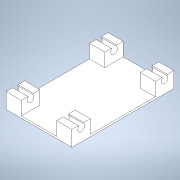
# Autodesk Inventor part: Kuka_base
Saved by Autodesk Inventor 2022 (Build 260153000, 153)
## iProperties
Created: 2022-08-12
Part Number: Kuka_base
Material: Generic
Document SubType Name: Modeling
Designer: Alok
Density: 1 g/cm^3
Appearance: Default
Author: Alok
Autodesk Inventor part; units mm, degrees
ref_plane "YZ Plane" through (0, 0, 0) normal (1, 0, 0) x (0, 1, 0)
ref_plane "XZ Plane" through (0, 0, 0) normal (0, 1, 0) x (-1, 0, 0)
ref_plane "XY Plane" through (0, 0, 0) normal (0, 0, 1) x (1, 0, 0)
sketch "Sketch1" plane through (0, 0, 0) normal (0, 1, 0) x (-1, 0, 0)
  line L0 (195, 302.5) -> (-195, 302.5)
  line L1 (-195, 302.5) -> (-195, -302.5)
  line L2 (-195, -302.5) -> (195, -302.5)
  line L3 (195, -302.5) -> (195, 302.5)
  line L4 (195, 302.5) -> (-195, -302.5) construction
  line L5 (-195, 302.5) -> (195, -302.5) construction
  point P0 (0, 0)
  dimension "d0" = 390
  dimension "d1" = 605
  constraints: 12 end point, 2 midpoint, 2 parallel, 1 horizontal, 1 perpendicular
  measures "d0" distance of L2.end L1.end
  measures "d1" distance of L1.end L0.end
extrude "Extrusion1" add sketch "Sketch1" along normal blind 12
sketch "Sketch2" plane through (0, 12, 0) normal (0, 1, 0) x (1, 0, 0)
  line L0 (-195, 302.5) -> (-195, -302.5) projected
  line L1 (-195, -302.5) -> (-195, -192.5)
  line L2 (-195, -302.5) -> (-85, -302.5) construction
  line L3 (-195, -192.5) -> (-105, -192.5)
  line L4 (-105, -192.5) -> (-105, -302.5)
  line L5 (-105, -302.5) -> (-195, -302.5)
  point P0 (0, 0)
  dimension "d4" = 110
  dimension "d5" = 90
  dimension "d6" = 90
  dimension "d7" = 90
  constraints: 10 end point, 4 perpendicular, 1 collinear, 1 horizontal
  measures "d4" distance of L0.end L1.end
  measures "d5" angle of L2 L1
  measures "d6" distance of L1.end L3.end
  measures "d7" angle of L1 L3
extrude "Extrusion2" add sketch "Sketch2" along normal blind 80
sketch "Sketch3" plane through (-195, 0, -302.5) normal (-1, 0, 0) x (0, 0, 1)
  line L0 (495, 92) -> (605, 92) projected
  line L1 (495, 92) -> (550, 92)
  line L2 (550, 92) -> (550, 73)
  line L3 (550, 92) -> (569, 92) construction
  circle A0 centre (550, 73) radius 20
  point P0 (302.5, 0)
  point P1 (543.755, 92)
  point P2 (556.245, 92)
  dimension "d10" = 55
  dimension "d11" = 19
  dimension "d12" = 90
  dimension "d13" = 40
  constraints: 6 end point, 1 centre point, 1 coincident, 1 horizontal, 1 midpoint, 1 perpendicular, 1 vertical
  measures "d10" distance of L0.start L1.end
  measures "d11" distance of L1.end L2.end
  measures "d12" angle of L2 L3
  measures "d13" diameter of A0
extrude "Extrusion3" cut sketch "Sketch3" against normal blind 110 contours L0 A0 picked at (549.7853, 66.101)
sketch "Sketch4" plane through (-195, 0, -302.5) normal (-1, 0, 0) x (0, 0, 1)
  line L0 (495, 92) -> (543.755, 92) projected
  line L1 (543.755, 92) -> (533.755, 92)
  line L2 (533.755, 92) -> (537.2905, 88.4645)
  arc A0 (543.755, 92) -> (556.245, 92) centre (550, 73) ccw projected
  line L3 (537.2905, 88.4645) -> (543.755, 92)
  point P0 (302.5, 0)
  dimension "d16" = 10
  dimension "d17" = 5
  dimension "d18" = 45
  constraints: 6 end point, 1 point on line
  measures "d16" distance of L0.end L1.end
  measures "d17" distance of L1.end L2.end
  measures "d18" angle of L2 L1
extrude "Extrusion4" cut sketch "Sketch4" against normal blind 110
sketch "Sketch5" plane through (-195, 0, -302.5) normal (-1, 0, 0) x (0, 0, 1)
  arc A0 (537.3715, 88.5088) -> (556.245, 92) centre (550, 73) ccw projected
  line L0 (556.245, 92) -> (566.245, 92)
  line L1 (556.245, 92) -> (605, 92) projected
  line L2 (556.245, 92) -> (566.245, 92) construction
  line L3 (566.245, 92) -> (562.7095, 88.4645)
  line L4 (562.7095, 88.4645) -> (556.245, 92)
  point P0 (302.5, 0)
  dimension "d21" = 10
  dimension "d22" = 0
  dimension "d23" = 5
  dimension "d24" = 45
  constraints: 8 end point, 2 collinear, 1 horizontal
  measures "d21" distance of L0.start L0.end
  measures "d22" distance between parallel lines of L0 L2
  measures "d23" distance of L0.end L3.end
  measures "d24" angle of L0 L3
extrude "Extrusion5" cut sketch "Sketch5" against normal blind 110
mirror "Mirror1" about plane through (0, 0, 0) normal (0, 0, 1) of "Extrusion2"
sketch "Sketch6" plane through (-105, 12, -302.5) normal (1, 0, 0) x (0, 0, -1)
  line L0 (-110, 80) -> (-55, 80)
  line L1 (0, 80) -> (-110, 80) projected
  line L2 (-55, 80) -> (-55, 61)
  circle A0 centre (-55, 61) radius 20
  point P0 (-302.5, -12)
  point P1 (-61.245, 80)
  point P2 (-48.755, 80)
  dimension "d27" = 55
  dimension "d28" = 19
  dimension "d29" = 40
  constraints: 4 end point, 1 centre point, 1 coincident, 1 midpoint, 1 vertical
  measures "d27" distance of L0.start L0.end
  measures "d28" distance of L0.end L2.end
  measures "d29" diameter of A0
extrude "Extrusion6" cut sketch "Sketch6" against normal blind 110 contours L0 L1 A0 picked at (-55.2147, 54.101)
mirror "Mirror2" about plane through (0, 0, 0) normal (1, 0, 0) of "Extrusion2", "Mirror1"
sketch "Sketch7" plane through (195, 0, 302.5) normal (1, 0, 0) x (0, 0, -1)
  arc A0 (543.755, 92) -> (556.245, 92) centre (550, 73) ccw projected
  circle A1 centre (550, 73) radius 20
  point P0 (302.5, 0)
  constraints: 1 centre point, 1 coincident
extrude "Extrusion7" cut sketch "Sketch7" against normal blind 110
sketch "Sketch8" plane through (195, 0, 302.5) normal (1, 0, 0) x (0, 0, -1)
  arc A0 (42.3715, 88.5088) -> (67.6285, 88.5088) centre (55, 73) ccw projected
  circle A1 centre (55, 73) radius 20
  point P0 (302.5, 0)
  point P1 (67.6285, 88.5088)
  constraints: 1 centre point, 1 coincident
extrude "Extrusion8" cut sketch "Sketch8" against normal blind 110
sketch "Sketch9" plane through (195, 0, 302.5) normal (1, 0, 0) x (0, 0, -1)
  line L0 (48.755, 92) -> (38.755, 92)
  line L1 (48.755, 92) -> (0, 92) projected
  line L2 (38.755, 92) -> (42.3026, 88.4524)
  arc A0 (48.755, 92) -> (61.245, 92) centre (55, 73) ccw projected
  line L3 (42.3026, 88.4524) -> (48.755, 92)
  point P0 (302.5, 0)
  dimension "d36" = 10
  dimension "d37" = 45
  constraints: 6 end point, 1 point on circle, 1 point on line
  measures "d36" distance of L0.start L0.end
  measures "d37" angle of L2 L0
extrude "Extrusion9" cut sketch "Sketch9" against normal blind 110
sketch "Sketch10" plane through (195, 0, 302.5) normal (1, 0, 0) x (0, 0, -1)
  arc A0 (42.3026, 88.4524) -> (61.245, 92) centre (55, 73) ccw projected
  line L0 (61.245, 92) -> (71.245, 92)
  line L1 (110, 92) -> (61.245, 92) projected
  line L2 (71.245, 92) -> (67.7095, 88.4645)
  line L3 (67.7095, 88.4645) -> (61.245, 92)
  point P0 (302.5, 0)
  dimension "d40" = 10
  dimension "d41" = 5
  dimension "d42" = 45
  constraints: 6 end point, 1 point on line
  measures "d40" distance of L0.start L0.end
  measures "d41" distance of L0.end L2.end
  measures "d42" angle of L0 L2
extrude "Extrusion10" cut sketch "Sketch10" against normal blind 110
sketch "Sketch11" plane through (195, 0, 302.5) normal (1, 0, 0) x (0, 0, -1)
  line L0 (543.755, 92) -> (495, 92) projected
  line L1 (543.755, 92) -> (533.755, 92)
  line L2 (533.755, 92) -> (537.2905, 88.4645)
  arc A0 (543.755, 92) -> (556.245, 92) centre (550, 73) ccw projected
  line L3 (537.2905, 88.4645) -> (543.755, 92)
  point P0 (302.5, 0)
  dimension "d45" = 10
  dimension "d46" = 5
  dimension "d47" = 45
  constraints: 6 end point, 1 point on line
  measures "d45" distance of L0.start L1.end
  measures "d46" distance of L1.end L2.end
  measures "d47" angle of L2 L1
extrude "Extrusion11" cut sketch "Sketch11" against normal blind 110
sketch "Sketch12" plane through (195, 0, 302.5) normal (1, 0, 0) x (0, 0, -1)
  line L0 (556.245, 92) -> (566.245, 92)
  line L1 (605, 92) -> (556.245, 92) projected
  line L2 (566.245, 92) -> (562.7095, 88.4645)
  arc A0 (537.3715, 88.5088) -> (556.245, 92) centre (550, 73) ccw projected
  line L3 (562.7095, 88.4645) -> (556.245, 92)
  point P0 (302.5, 0)
  dimension "d50" = 10
  dimension "d51" = 5
  dimension "d52" = 45
  constraints: 6 end point, 1 point on line
  measures "d50" distance of L0.start L0.end
  measures "d51" distance of L0.end L2.end
  measures "d52" angle of L0 L2
extrude "Extrusion12" cut sketch "Sketch12" against normal blind 110
sketch "Sketch13" plane through (-195, 0, -302.5) normal (-1, 0, 0) x (0, 0, 1)
  line L0 (0, 92) -> (48.755, 92) projected
  line L1 (48.755, 92) -> (38.755, 92)
  line L2 (38.755, 92) -> (42.2905, 88.4645)
  line L3 (42.2905, 88.4645) -> (48.755, 92)
  line L4 (61.245, 92) -> (110, 92) projected
  line L5 (61.245, 92) -> (71.245, 92)
  line L6 (71.245, 92) -> (67.7095, 88.4645)
  arc A0 (48.755, 92) -> (61.245, 92) centre (55, 73) ccw projected
  line L7 (67.7095, 88.4645) -> (61.245, 92)
  point P0 (302.5, 0)
  dimension "d55" = 10
  dimension "d56" = 5
  dimension "d57" = 45
  dimension "d58" = 10
  dimension "d59" = 5
  dimension "d60" = 45
  constraints: 12 end point, 2 point on line, 1 perpendicular
  measures "d55" distance of L0.end L1.end
  measures "d56" distance of L1.end L2.end
  measures "d57" angle of L2 L1
  measures "d58" distance of L4.start L5.end
  measures "d59" distance of L5.end L6.end
  measures "d60" angle of L5 L6
extrude "Extrusion13" cut sketch "Sketch13" against normal blind 110
body "Solid1"
